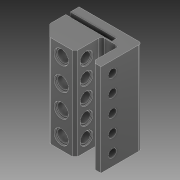
# Autodesk Inventor part: Chain Clamp (3DP)
Saved by Autodesk Inventor 2021 (Build 250183000, 183)
## iProperties
Created: 2020-09-06
Part Number: Chain Clamp (3DP)
Material: Nylon 6/6
Document SubType Name: Modeling
Density: 1.13 g/cm^3
Appearance: Smooth - Black
Autodesk Inventor part; units mm, degrees
ref_plane "YZ Plane" through (0, 0, 0) normal (1, 0, 0) x (0, 1, 0)
ref_plane "XZ Plane" through (0, 0, 0) normal (0, 1, 0) x (-1, 0, 0)
sketch "Sketch1" plane through (0, 0, 0) normal (0, 1, 0) x (-1, 0, 0)
  line L0 (0, 0) -> (17.145, 0)
  line L1 (17.145, 0) -> (17.145, 15.24)
  line L2 (17.145, 15.24) -> (0, 15.24)
  line L3 (0, 15.24) -> (0, 0)
  line L4 (0, 15.24) -> (-3.175, 15.24)
  line L5 (-3.175, 15.24) -> (-3.175, -2.54)
  line L6 (-3.175, -2.54) -> (0, -2.54)
  line L7 (0, -2.54) -> (0, 15.24)
  line L8 (-3.175, -2.54) -> (-12.7, -2.54)
  line L9 (-12.7, -2.54) -> (-12.7, 0.635)
  line L10 (-12.7, 0.635) -> (-3.175, 0.635)
  line L11 (-3.175, 0.635) -> (-3.175, -2.54)
  line L12 (-12.7, -2.54) -> (-17.4625, -2.54)
  line L13 (-17.4625, -2.54) -> (-17.4625, 15.24)
  line L14 (-17.4625, 15.24) -> (-12.7, 15.24)
  line L15 (-12.7, 15.24) -> (-12.7, -2.54)
  line L16 (0, -2.54) -> (-17.4625, -2.54)
  line L17 (-17.4625, -2.54) -> (-17.4625, -7.3025)
  line L18 (-17.4625, -7.3025) -> (0, -7.3025)
  line L19 (0, -7.3025) -> (0, -2.54)
  line L20 (0, 0) -> (-3.175, 0)
  line L21 (0, -2.54) -> (17.145, -2.54)
  line L22 (17.145, -2.54) -> (17.145, -7.3025)
  line L23 (17.145, -7.3025) -> (0, -7.3025)
  line L24 (0, -7.3025) -> (0, -2.54)
  line L25 (17.145, -2.54) -> (-8.255, -2.54)
  line L26 (-8.255, -2.54) -> (-8.255, 0)
  line L27 (-8.255, 0) -> (17.145, 0)
  line L28 (17.145, 0) -> (17.145, -2.54)
  point P0 (0, 0)
  point P1 (-3.175, 0.635)
  point P2 (-12.7, 0.635)
  point P3 (0, 0)
  point P4 (-3.175, 0)
  dimension "d0" = 2.54
  dimension "d1" = 15.24
  dimension "d2" = 17.145
  dimension "d3" = 4.7625
  dimension "d4" = 9.525
  dimension "d5" = 3.175
  dimension "d6" = 3.175
  dimension "d34" = 4.7625
  dimension "d61" = 25.4
  constraints: 58 end point, 14 parallel, 8 perpendicular, 7 horizontal, 3 collinear, 2 point on line, 1 coincident
  measures "d0" distance between parallel lines of L8 L0
  measures "d1" distance between parallel lines of L2 L0
  measures "d2" distance between parallel lines of L7 L1
  measures "d3" distance between parallel lines of L15 L13
  measures "d4" distance between parallel lines of L15 L5
  measures "d5" distance between parallel lines of L8 L10
  measures "d6" distance between parallel lines of L7 L5
  measures "d34" distance of L12.end L17.end
  measures "d61" distance of L26.end L27.end
extrude "Extrusion1" add sketch "Sketch1" along normal blind 50.8 contours L3 L2 L1 L0 | L20 L5 L4 L3 | L19 L18 L17 L12 L8 L6 | L21 L22 L23 L19 | L27 L26 L8 L9 L10 L5 | L9 L12 L13 L14 L15
sketch "Sketch2" plane through (-17.145, 0, 15.24) normal (0, 0, 1) x (1, 0, 0)
  line L0 (0, 0) -> (20.32, 0) projected
  line L1 (20.32, 0) -> (20.32, 50.8) projected
  line L2 (0, 50.8) -> (20.32, 50.8) projected
  line L3 (0, 0) -> (0, 50.8) projected
  circle A0 centre (12.7, 6.35) radius 2.4892
  circle A1 centre (12.7, 19.05) radius 2.4892
  circle A2 centre (12.7, 31.75) radius 2.4892
  circle A3 centre (12.7, 44.45) radius 2.4892
  point P0 (17.145, 0)
  dimension "d9" = 4.9784
  dimension "d12" = 12.7
  dimension "d17" = 6.35
  dimension "d43" = 12.7
  constraints: 4 centre point, 4 coincident, 1 vertical, 9 other
  measures "d9" diameter of A0
  measures "d12" distance of point (12.7, 6.35) point (12.7, 19.05)
  measures "d17" distance from line of L2 point (12.7, 44.45)
  measures "d43" distance from line of L3 point (12.7, 6.35)
extrude "Extrusion2" cut sketch "Sketch2" against normal blind 50.8 contours A0 | A1 | A2 | A3
sketch "Sketch3" plane through (17.4625, 0, 15.24) normal (1, 0, 0) x (0, 0, -1)
  line L0 (6.35, 0.3715) -> (6.35, 6.35)
  circle A0 centre (6.35, 6.35) radius 2.2479
  circle A1 centre (6.35, 15.875) radius 2.2479
  circle A2 centre (6.35, 25.4) radius 2.2479
  circle A3 centre (6.35, 34.925) radius 2.2479
  circle A4 centre (6.35, 44.45) radius 2.2479
  line L1 (0, 50.8) -> (22.5425, 50.8) projected
  line L2 (0, 0) -> (0, 50.8) projected
  dimension "d21" = 4.4958
  dimension "d24" = 9.525
  dimension "d51" = 6.35
  dimension "d60" = 6.35
  constraints: 5 centre point, 5 coincident, 2 end point, 2 vertical, 12 other
  measures "d21" diameter of A0
  measures "d24" distance of L0.end point (6.35, 15.875)
  measures "d51" distance from line of L1 point (6.35, 44.45)
  measures "d60" distance from line of L2 L0.end
extrude "Extrusion3" cut sketch "Sketch3" against normal blind 9.525
chamfer "Chamfer1" distance 6.35 angle 45 1 edges at (-17.145, 25.4, 15.24)
chamfer "Chamfer2" distance 1.5875 angle 45 2 edges at (3.175, 25.4, 15.24) (12.7, 25.4, 15.24)
fillet "Fillet1" radius 1.5875 5 edges at (12.7, 25.4, 0.635) (3.175, 25.4, 0.635) (17.4625, 25.4, -7.3025) (-17.145, 25.4, 8.89) (-10.795, 25.4, 15.24)
sketch "Sketch4" plane through (1.5875, 0, 15.24) normal (0, 0, 1) x (1, 0, 0)
  circle A0 centre (-6.0325, 44.45) radius 2.4892 projected
  circle A1 centre (-6.0325, 31.75) radius 2.4892 projected
  circle A2 centre (-6.0325, 19.05) radius 2.4892 projected
  circle A3 centre (-6.0325, 6.35) radius 2.4892 projected
  point P0 (-1.5875, 0)
  constraints: 4 coincident
hole "Hole1" at (-4.445, 44.45, 15.24) at (-4.445, 31.75, 15.24) at (-4.445, 19.05, 15.24) at (-4.445, 6.35, 15.24) direction (0, 0, -1) diameter 6.35 depth 9.525 counterbore diameter 7.9375 counterbore depth 1.016
ref_plane "Work Plane1" through (3.175, 0, 15.24) normal (1, 0, 0) x (0, 0, -1)
sketch "Sketch5" plane through (3.175, 0, 15.24) normal (1, 0, 0) x (0, 0, -1)
  line L0 (20.955, 50.8) -> (20.955, 0) projected
  line L1 (0, 50.8) -> (20.955, 50.8) projected
  line L2 (0, 0) -> (0, 50.8) projected
  line L3 (0, 0) -> (20.955, 0) projected
  circle A0 centre (6.35, 25.4) radius 2.2479 projected
  circle A1 centre (6.35, 15.875) radius 2.2479 projected
  circle A2 centre (6.35, 34.925) radius 2.2479 projected
  circle A3 centre (6.35, 6.35) radius 2.2479 projected
  circle A4 centre (6.35, 44.45) radius 2.2479 projected
  point P0 (15.24, 0)
hole "Hole2" at (3.175, 44.45, 8.89) at (3.175, 34.925, 8.89) at (3.175, 25.4, 8.89) at (3.175, 15.875, 8.89) at (3.175, 6.35, 8.89) direction (-1, 0, 0) diameter 5.588 depth 7.9375 counterbore diameter 7.112 counterbore depth 0.762
equation "\"d31\" = d24"
body "Solid1"
